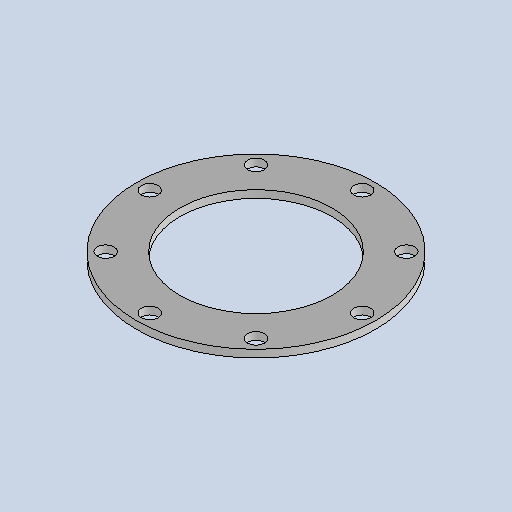
# Autodesk Inventor part: TKS 3001 BOTTOM DS main flange
Saved by Autodesk Inventor 2025.1 (Build 291241020, 241B)
## iProperties
Created: 2024-12-09
Part Number: TKS 3001 BOTTOM DS main flange
Material: Stainless Steel
Document SubType Name: Sheet Metal
Designer: user
Mass: 3269.02 g
Surface Area: 1007.63 cm^2
Volume: 408.627 cm^3
Density: 8 g/cm^3
Flat Pattern Width: 31.5 cm
Flat Pattern Length: 31.5 cm
Flat Pattern Area: 992.25 cm^2
Sheet Metal Rule: AISI304 3mm Die 32
Sheet Metal Width: 315.000 mm
Sheet Metal Length: 315.000 mm
Sheet Metal Area: 99225.000 mm^2
Appearance: Default
Author: user
Autodesk Inventor part; units mm, degrees
ref_plane "YZ Plane" through (0, 0, 0) normal (1, 0, 0) x (0, 1, 0)
ref_plane "XZ Plane" through (0, 0, 0) normal (0, 1, 0) x (-1, 0, 0)
ref_plane "XY Plane" through (0, 0, 0) normal (0, 0, 1) x (1, 0, 0)
sketch "Sketch1" plane through (0, 0, 0) normal (0, 0, 1) x (1, 0, 0)
  circle A0 centre (0, 0) radius 100
  circle A1 centre (0, 0) radius 157.5
  dimension "d22" = 200
  dimension "d23" = 315
  measures "d22" diameter of A0
  measures "d23" diameter of A1
extrude "Plate1" add sketch "Sketch1" along normal blind 10
sketch "Sketch5" plane through (0, 0, 10) normal (0, 0, 1) x (1, 0, 0)
  circle A0 centre (0, 140) radius 11
  circle A1 centre (0, 0) radius 140 construction
  dimension "d25" = 280
  dimension "d24" = 22
  constraints: 2 vertical alignment, 1 centre point, 1 coincident, 2 other
  measures "d24" diameter of A0
extrude "Cut1" cut sketch "Sketch5" against normal blind 10
pattern_circular "Circular Pattern1" count 8 over 360 about axis through (0, 0, 0) along (0, 0, 1) of "Cut1"
equation "\"d26\" = Thickness"
equation "\"d2\" = Thickness"
equation "\"BendReliefDepth\" = 0.5 * Thickness"
equation "\"TransitionRadius\" = BendRadius"
equation "\"JacobiRadiusSize\" = BendRadius"
equation "\"Thickness\" = 10"
equation "\"BendRadius\" = 5"
body "Solid1"
